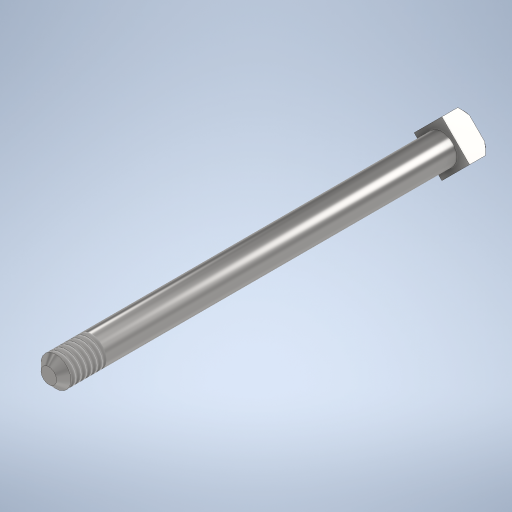
# Autodesk Inventor part: ES117_Bolt
Saved by Autodesk Inventor 2024 (Build 280153000, 153)
## iProperties
Created: 2023-06-04
Part Number: ES117_Bolt
Material: Stainless Steel
Document SubType Name: Modeling
Designer: vilas
Density: 8 g/cm^3
Appearance: Semi-Polished
Author: vilas
Autodesk Inventor part; units mm, degrees
ref_plane "YZ Plane" through (0, 0, 0) normal (1, 0, 0) x (0, 1, 0)
ref_plane "XZ Plane" through (0, 0, 0) normal (0, 1, 0) x (-1, 0, 0)
ref_plane "XY Plane" through (0, 0, 0) normal (0, 0, 1) x (1, 0, 0)
sketch "Sketch1" plane through (0, 0, 0) normal (0, 0, 1) x (1, 0, 0)
  line L0 (-3.8891, 0) -> (0, -3.8891)
  line L1 (0, -3.8891) -> (3.8891, 0)
  line L2 (3.8891, 0) -> (0, 3.8891)
  line L3 (0, 3.8891) -> (-3.8891, 0)
  line L4 (-3.8891, 0) -> (3.8891, 0) construction
  line L5 (0, -3.8891) -> (0, 3.8891) construction
  point P0 (0, 0)
  dimension "d0" = 5.5
  dimension "d1" = 5.5
  dimension "d2" = 90
  dimension "d3" = 5.5
  dimension "d4" = 90
  dimension "d5" = 0
  dimension "d6" = 0
  constraints: 12 end point, 2 perpendicular, 1 horizontal, 1 vertical
  measures "d0" distance of L0.start L0.end
  measures "d1" distance of L0.end L1.end
  measures "d2" angle of L1 L0
  measures "d3" distance of L1.end L2.end
  measures "d4" angle of L2 L1
  measures "d5" distance from line of point (0, 0) L4
  measures "d6" distance from line of point (0, 0) L5
extrude "Extrusion1" add sketch "Sketch1" along normal blind 3
sketch "Sketch2" plane through (0, 0, 0) normal (1, 0, 0) x (0, 1, 0)
  line L0 (3.8891, 0) -> (0, 0) projected
  line L1 (3.8891, 0) -> (3.8891, 0.75)
  line L2 (3.8891, 0.75) -> (3.1391, 0)
  line L3 (3.8891, 0) -> (3.1391, 0)
  line L4 (-3.8891, 3) -> (0, 3) projected
  line L5 (0, 3) -> (0, 0)
  dimension "d9" = 0.75
  dimension "d10" = 0.75
  constraints: 8 end point, 1 collinear, 1 perpendicular, 1 point on line, 1 vertical
  measures "d9" distance of L0.start L1.end
  measures "d10" distance of L2.end L0.start
revolve "Revolution1" cut sketch "Sketch2" angle 360 about axis through (0, 0, 3) along (0, 0, -1)
sketch "Sketch3" plane through (0, 0, 3) normal (0, 0, 1) x (1, 0, 0)
  circle A0 centre (0, 0) radius 2.1
  dimension "d12" = 4.2
  constraints: 1 centre point, 1 coincident
  measures "d12" diameter of A0
extrude "Extrusion2" add sketch "Sketch3" along normal blind 55.206
chamfer "Chamfer1" distance 1 angle 45 1 edges at (-2.1, 0, 58.206)
thread "Thread1" size "M4.5x0.75" class "6g" standard "ANSI Metric M Profile" length 5
body "Solid1"
